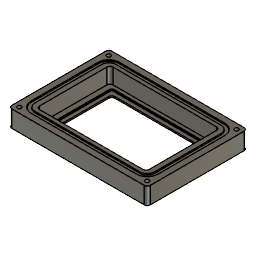
Base V3.4 (Autodesk Fusion 360 design; units mm, degrees)
part number: 2026-01-30-14-30-51-369
Autodesk Fusion 360 part; units mm, degrees
note: some values were not read from the file. Set by a fixed rule: which sketch regions a step uses.
sketch "Sketch1" plane through (0, 0, 0) normal (0, 0, 1) x (1, 0, 0)
  line L0 (86, -65) -> (-86, -65)
  line L1 (-90, -61) -> (-90, 61)
  line L2 (-86, 65) -> (86, 65)
  line L3 (90, 61) -> (90, -61)
  line L4 (90, -65) -> (-90, 65) construction
  line L5 (-90, -65) -> (90, 65) construction
  arc A0 (-86, 65) -> (-90, 61) centre (-86, 61) ccw
  arc A1 (90, 61) -> (86, 65) centre (86, 61) ccw
  arc A2 (86, -65) -> (90, -61) centre (86, -61) ccw
  arc A3 (-90, -61) -> (-86, -65) centre (-86, -61) ccw
  circle A4 centre (-83, 58) radius 2.6
  line L6 (0, 65) -> (0, -65) construction
  line L7 (90, 0) -> (-90, 0) construction
  circle A5 centre (83, 58) radius 2.6
  circle A6 centre (83, -58) radius 2.6
  circle A7 centre (-83, -58) radius 2.6
  dimension "d1" = 180
  dimension "d2" = 130
  dimension "d26" = 4
  dimension "d27" = 4
  dimension "d28" = 4
  dimension "d29" = 4
  dimension "d30" = 5.2
  dimension "d31" = 7
  dimension "d32" = 7
  constraint horizontal L0
  constraint perpendicular L0 L1
  constraint parallel L0 L2
  constraint parallel L1 L3
  constraint coincident L4 origin
  constraint coincident L5 origin
  constraint coincident L4.end L2
  constraint coincident L4.end L1
  constraint tangent L2 A0
  constraint tangent L1 A0
  constraint coincident L5.end L3
  constraint coincident L5.end L2
  constraint tangent L3 A1
  constraint tangent L2 A1
  constraint coincident L4.start L3
  constraint coincident L4.start L0
  constraint tangent L3 A2
  constraint tangent L0 A2
  constraint coincident L5.start L1
  constraint coincident L5.start L0
  constraint tangent L1 A3
  constraint tangent L0 A3
  constraint midpoint L2 L6.start
  constraint midpoint L0 L6.end
  constraint midpoint L3 L7.start
  constraint midpoint L1 L7.end
  constraint symmetric A4 L6 A5
  constraint symmetric A4 L7 A7
  constraint symmetric L7 A5 A6
  measures "d1" distance of L4.end L5.end
  measures "d2" distance of L5.start L4.end
  measures "d26" radius of A0
  measures "d27" radius of A1
  measures "d28" radius of A2
  measures "d29" radius of A3
  measures "d30" diameter of A4
  measures "d31" distance of L2 A4.centre
  measures "d32" distance of L1 A4.centre
extrude "Extrude1" add sketch "Sketch1" along normal blind 22
sketch "Sketch2" plane through (0, 0, 22) normal (0, 0, 1) x (-1, 0, 0)
  line L0 (-86, -65) -> (86, -65)
  line L1 (90, -61) -> (90, 61)
  line L2 (86, 65) -> (-86, 65)
  line L3 (-90, 61) -> (-90, -61)
  line L4 (-67.2, 47.75) -> (67.2, 47.75)
  line L5 (71.2, 43.75) -> (71.2, -43.75)
  line L6 (67.2, -47.75) -> (-67.2, -47.75)
  line L7 (-71.2, -43.75) -> (-71.2, 43.75)
  line L8 (-71.2, 47.75) -> (71.2, -47.75) construction
  line L9 (71.2, 47.75) -> (-71.2, -47.75) construction
  arc A0 (86, -65) -> (90, -61) centre (86, -61) ccw
  arc A1 (90, 61) -> (86, 65) centre (86, 61) ccw
  arc A2 (-86, 65) -> (-90, 61) centre (-86, 61) ccw
  arc A3 (-90, -61) -> (-86, -65) centre (-86, -61) ccw
  circle A4 centre (83, 58) radius 2.6
  circle A5 centre (-83, 58) radius 2.6
  circle A6 centre (-83, -58) radius 2.6
  circle A7 centre (83, -58) radius 2.6
  arc A8 (67.2, -47.75) -> (71.2, -43.75) centre (67.2, -43.75) ccw
  arc A9 (-71.2, -43.75) -> (-67.2, -47.75) centre (-67.2, -43.75) ccw
  arc A10 (71.2, 43.75) -> (67.2, 47.75) centre (67.2, 43.75) ccw
  arc A11 (-67.2, 47.75) -> (-71.2, 43.75) centre (-67.2, 43.75) ccw
  dimension "d5" = 142.4
  dimension "d6" = 95.5
  dimension "d52" = 4
  dimension "d53" = 4
  dimension "d54" = 4
  dimension "d55" = 4
  constraint horizontal L4
  constraint perpendicular L4 L5
  constraint parallel L4 L6
  constraint parallel L5 L7
  constraint coincident L8 origin
  constraint coincident L9 origin
  constraint coincident L8.end L6
  constraint coincident L8.end L5
  constraint tangent L6 A8
  constraint tangent L5 A8
  constraint coincident L9.end L6
  constraint coincident L9.end L7
  constraint tangent L6 A9
  constraint tangent L7 A9
  constraint coincident L9.start L5
  constraint coincident L9.start L4
  constraint tangent L5 A10
  constraint tangent L4 A10
  constraint coincident L8.start L7
  constraint coincident L8.start L4
  constraint tangent L7 A11
  constraint tangent L4 A11
  measures "d5" distance of L8.end L9.end
  measures "d6" distance of L9.start L8.end
  measures "d52" radius of A8
  measures "d53" radius of A9
  measures "d54" radius of A10
  measures "d55" radius of A11
extrude "Extrude2" cut sketch "Sketch2" against normal blind 20 contours L4 L5 L6 L7 A8 A9 A10 A11
sketch "Sketch3" plane through (0, 0, 22) normal (0, 0, 1) x (-1, 0, 0)
  line L0 (71.2, 43.75) -> (71.2, -43.75)
  line L1 (67.2, -47.75) -> (-67.2, -47.75)
  line L2 (-71.2, -43.75) -> (-71.2, 43.75)
  line L3 (-67.2, 47.75) -> (67.2, 47.75)
  line L4 (-86, -65) -> (86, -65)
  line L5 (90, -61) -> (90, 61)
  line L6 (86, 65) -> (-86, 65)
  line L7 (-90, 61) -> (-90, -61)
  line L8 (-79.9494, 54.9494) -> (79.9494, 54.9494) construction
  line L9 (79.9494, 54.9494) -> (79.9494, -54.9494) construction
  line L10 (79.9494, -54.9494) -> (-79.9494, -54.9494) construction
  line L11 (-79.9494, -54.9494) -> (-79.9494, 54.9494) construction
  line L12 (-79.9494, 54.9494) -> (79.9494, -54.9494) construction
  line L13 (79.9494, 54.9494) -> (-79.9494, -54.9494) construction
  line L14 (77.8149, 43.2459) -> (77.8149, -43.2459)
  line L15 (68.2459, -52.8149) -> (-68.2459, -52.8149)
  line L16 (-77.8149, -43.2459) -> (-77.8149, 43.2459)
  line L17 (-69.6267, 47.2574) -> (77.8149, -52.8149) construction
  line L18 (70.6619, 45.6619) -> (-70.6619, -45.6619) construction
  line L19 (-68.2459, 57.0839) -> (68.2459, 57.0839)
  line L20 (82.0839, 43.2459) -> (82.0839, -43.2459)
  line L21 (68.2459, -57.0839) -> (-68.2459, -57.0839)
  line L22 (-82.0839, -43.2459) -> (-82.0839, 43.2459)
  line L23 (-72.3401, 50.3077) -> (82.0839, -57.0839) construction
  line L24 (73.5309, 48.5309) -> (-73.5309, -48.5309) construction
  arc A0 (68.2459, -52.8149) -> (77.8149, -43.2459) centre (68.2459, -43.2459) ccw
  arc A1 (68.2459, -57.0839) -> (82.0839, -43.2459) centre (68.2459, -43.2459) ccw
  line L25 (0, -65) -> (0, 65) construction
  line L26 (-90, 0) -> (90, 0) construction
  arc A2 (-77.8149, -43.2459) -> (-68.2459, -52.8149) centre (-68.2459, -43.2459) ccw
  arc A3 (-82.0839, -43.2459) -> (-68.2459, -57.0839) centre (-68.2459, -43.2459) ccw
  arc A4 (-68.2459, 52.8149) -> (-77.8149, 43.2459) centre (-68.2459, 43.2459) ccw
  arc A5 (-68.2459, 57.0839) -> (-82.0839, 43.2459) centre (-68.2459, 43.2459) ccw
  arc A6 (77.8149, 43.2459) -> (68.2459, 52.8149) centre (68.2459, 43.2459) ccw
  arc A7 (82.0839, 43.2459) -> (68.2459, 57.0839) centre (68.2459, 43.2459) ccw
  line L27 (-68.2459, 52.8149) -> (68.2459, 52.8149)
  arc A8 (86, -65) -> (90, -61) centre (86, -61) ccw
  arc A9 (90, 61) -> (86, 65) centre (86, 61) ccw
  arc A10 (-86, 65) -> (-90, 61) centre (-86, 61) ccw
  arc A11 (-90, -61) -> (-86, -65) centre (-86, -61) ccw
  circle A12 centre (83, 58) radius 2.6
  circle A13 centre (-83, 58) radius 2.6
  circle A14 centre (-83, -58) radius 2.6
  circle A15 centre (83, -58) radius 2.6
  arc A16 (71.2, 43.75) -> (67.2, 47.75) centre (67.2, 43.75) ccw
  arc A17 (67.2, -47.75) -> (71.2, -43.75) centre (67.2, -43.75) ccw
  arc A18 (-71.2, -43.75) -> (-67.2, -47.75) centre (-67.2, -43.75) ccw
  arc A19 (-67.2, 47.75) -> (-71.2, 43.75) centre (-67.2, 43.75) ccw
  dimension "d9" = 159.8988
  dimension "d15" = 109.8988
  dimension "d16" = 2.1345
  dimension "d17" = 2.1345
  dimension "d18" = 2.1345
  dimension "d19" = 2.1345
  dimension "d20" = 9.569
  dimension "d21" = 13.838
  constraint horizontal L8
  constraint perpendicular L8 L9
  constraint parallel L8 L10
  constraint parallel L9 L11
  constraint coincident L12 origin
  constraint coincident L13 origin
  constraint parallel L15 L27
  constraint parallel L14 L16
  constraint coincident L17 origin
  constraint coincident L18 origin
  constraint horizontal L19
  constraint perpendicular L19 L20
  constraint parallel L19 L21
  constraint parallel L20 L22
  constraint coincident L23 origin
  constraint coincident L24 origin
  constraint coincident L17.end L15
  constraint coincident L17.end L14
  constraint tangent L15 A0
  constraint tangent L14 A0
  constraint coincident L23.end L21
  constraint coincident L23.end L20
  constraint tangent L21 A1
  constraint tangent L20 A1
  constraint midpoint L4 L25.start
  constraint midpoint L6 L25.end
  constraint midpoint L7 L26.start
  constraint midpoint L5 L26.end
  constraint symmetric L15.start L25 L15.end
  constraint symmetric L14.end L25 L16.start
  constraint symmetric A0 L25 A2
  constraint symmetric L21.start L25 L21.end
  constraint symmetric L20.end L25 L22.start
  constraint symmetric A1 L25 A3
  constraint symmetric L15.start L26 A6.end
  constraint symmetric L14.end L26 L14.start
  constraint symmetric A0 L26 A6
  constraint symmetric L21.start L26 L19.end
  constraint symmetric L20.end L26 L20.start
  constraint symmetric A1 L26 A7
  constraint symmetric L26 L15.end A4.start
  constraint symmetric L26 L16.start L16.end
  constraint symmetric L26 A2 A4
  constraint symmetric L26 L21.end L19.start
  constraint symmetric L26 L22.start L22.end
  constraint symmetric L26 A3 A5
  measures "d9" distance of L8.start L8.end
  measures "d15" distance of L8 L10
  measures "d16" distance of L11 L16
  measures "d17" distance of L10 L15
  measures "d18" distance of L11 L22
  measures "d19" distance of L10 L21
  measures "d20" radius of A0
  measures "d21" radius of A1
extrude "Extrude3" cut sketch "Sketch3" against normal blind 1.424 contours L19 L20 L21 L22 A1 A3 A5 A7
draft "Draft1" angle 10 neutral plane through (0, 0, 20.576) pull (0, 0, 1) 16 faces at (-77.8149, -14.4153, 21.5253) (-71.8024, 52.1295, 21.0507) (-22.7486, 52.8149, 21.5253) (72.6307, 51.7512, 21.0507) (77.8149, 14.4153, 21.5253) (73.0304, -51.5329, 21.0507) (22.7486, -52.8149, 21.5253) (-77.1295, -46.8024, 21.0507) (-82.0839, -14.4153, 21.5253) (-76.2727, -54.518, 21.0507) (-22.7486, -57.0839, 21.0507) (82.0213, -44.5613, 21.0507) (82.0839, 14.4153, 21.5253) (77.7952, 53.2609, 21.0507) (22.7486, 57.0839, 21.0507) (-76.8, 54.1233, 21.0507)
sketch "Sketch6" plane through (0, 0, 2) normal (0, 0, 1) x (-1, 0, 0)
  arc A0 (71.2, 43.75) -> (67.2, 47.75) centre (67.2, 43.75) ccw
  line L0 (67.2, 47.75) -> (-67.2, 47.75)
  arc A1 (-67.2, 47.75) -> (-71.2, 43.75) centre (-67.2, 43.75) ccw
  line L1 (-71.2, 43.75) -> (-71.2, -43.75)
  arc A2 (-71.2, -43.75) -> (-67.2, -47.75) centre (-67.2, -43.75) ccw
  line L2 (-67.2, -47.75) -> (67.2, -47.75)
  arc A3 (67.2, -47.75) -> (71.2, -43.75) centre (67.2, -43.75) ccw
  line L3 (71.2, -43.75) -> (71.2, 43.75)
  arc A4 (60.9079, -41.3399) -> (62.4799, -39.7679) centre (60.9079, -39.7679) ccw construction
  arc A5 (-62.4799, -39.7399) -> (-60.9079, -41.3119) centre (-60.9079, -39.7399) ccw construction
  line L4 (-48.9575, -41.8399) -> (48.9575, -41.8399) construction
  line L5 (48.9575, 41.8399) -> (-48.9575, 41.8399) construction
  line L6 (-62.9799, 29.7119) -> (-62.9799, 27.8175) construction
  line L7 (48.9575, -41.8399) -> (50.8519, -41.8399) construction
  line L8 (62.4799, 30.3078) -> (62.4799, 39.7679) construction
  arc A6 (-60.88, 42.74) -> (-63.88, 39.74) centre (-60.88, 39.74) ccw construction
  line L9 (63.88, 39.74) -> (63.88, -39.74) construction
  arc A7 (63.88, 39.74) -> (60.88, 42.74) centre (60.88, 39.74) ccw construction
  line L10 (-62.9799, -29.7119) -> (-62.4799, -30.3078) construction
  line L11 (51.4478, 41.3399) -> (50.8519, 41.8399) construction
  arc A8 (60.88, -42.74) -> (63.88, -39.74) centre (60.88, -39.74) ccw construction
  line L12 (-48.9575, 41.8399) -> (-50.8519, 41.8399) construction
  line L13 (-60.88, 42.74) -> (60.88, 42.74) construction
  line L14 (-62.9799, -27.8175) -> (-62.9799, -29.7119) construction
  line L15 (60.88, -42.74) -> (-60.88, -42.74) construction
  line L16 (62.9799, 29.7119) -> (62.4799, 30.3078) construction
  line L17 (-50.8519, 41.8399) -> (-51.4811, 41.3119) construction
  line L18 (62.4799, -39.7679) -> (62.4799, -30.3078) construction
  line L19 (-50.8519, -41.8399) -> (-48.9575, -41.8399) construction
  line L20 (60.9079, 41.3399) -> (51.4478, 41.3399) construction
  line L21 (50.8519, 41.8399) -> (48.9575, 41.8399) construction
  line L22 (62.9799, 27.8175) -> (62.9799, 29.7119) construction
  line L23 (51.4478, -41.3399) -> (60.9079, -41.3399) construction
  line L24 (62.9799, -27.8175) -> (62.9799, 27.8175) construction
  line L25 (-63.88, -39.74) -> (-63.88, 39.74) construction
  line L26 (50.8519, -41.8399) -> (51.4478, -41.3399) construction
  line L27 (62.9799, -29.7119) -> (62.9799, -27.8175) construction
  arc A9 (-63.88, -39.74) -> (-60.88, -42.74) centre (-60.88, -39.74) ccw construction
  arc A10 (62.4799, 39.7679) -> (60.9079, 41.3399) centre (60.9079, 39.7679) ccw construction
  line L28 (62.4799, -30.3078) -> (62.9799, -29.7119) construction
  line L29 (-62.4799, 30.3078) -> (-62.9799, 29.7119) construction
  line L30 (-60.9079, -41.3119) -> (-51.4811, -41.3119) construction
  arc A11 (-60.9079, 41.3119) -> (-62.4799, 39.7399) centre (-60.9079, 39.7399) ccw construction
  line L31 (-51.4811, -41.3119) -> (-50.8519, -41.8399) construction
  line L32 (-51.4811, 41.3119) -> (-60.9079, 41.3119) construction
  line L33 (-62.4799, 39.7399) -> (-62.4799, 30.3078) construction
  line L34 (-62.4799, -30.3078) -> (-62.4799, -39.7399) construction
  line L35 (-62.9799, 27.8175) -> (-62.9799, -27.8175) construction
  line L36 (0, -47.75) -> (0, 47.75) construction
  line L37 (-71.2, 0) -> (71.2, 0) construction
  line L38 (-60.85, 43.25) -> (60.85, 43.25)
  line L39 (64.35, 39.75) -> (64.35, -39.75)
  line L40 (60.85, -43.25) -> (-60.85, -43.25)
  line L41 (-64.35, -39.75) -> (-64.35, 39.75)
  line L42 (-64.35, 43.25) -> (64.35, -43.25) construction
  line L43 (64.35, 43.25) -> (-64.35, -43.25) construction
  arc A12 (60.85, -43.25) -> (64.35, -39.75) centre (60.85, -39.75) ccw
  arc A13 (-64.35, -39.75) -> (-60.85, -43.25) centre (-60.85, -39.75) ccw
  arc A14 (-60.85, 43.25) -> (-64.35, 39.75) centre (-60.85, 39.75) ccw
  arc A15 (64.35, 39.75) -> (60.85, 43.25) centre (60.85, 39.75) ccw
  line L44 (-60.85, 40.75) -> (60.85, 40.75)
  line L45 (61.85, 39.75) -> (61.85, -39.75)
  line L46 (60.85, -40.75) -> (-60.85, -40.75)
  line L47 (-61.85, -39.75) -> (-61.85, 39.75)
  line L48 (-61.85, 40.75) -> (61.85, -40.75) construction
  line L49 (61.85, 40.75) -> (-61.85, -40.75) construction
  arc A16 (-61.85, -39.75) -> (-60.85, -40.75) centre (-60.85, -39.75) ccw
  arc A17 (60.85, -40.75) -> (61.85, -39.75) centre (60.85, -39.75) ccw
  arc A18 (61.85, 39.75) -> (60.85, 40.75) centre (60.85, 39.75) ccw
  arc A19 (-60.85, 40.75) -> (-61.85, 39.75) centre (-60.85, 39.75) ccw
  dimension "d56" = 128.7
  dimension "d57" = 86.5
  dimension "d58" = 3.5
  dimension "d59" = 3.5
  dimension "d60" = 3.5
  dimension "d61" = 3.5
  dimension "d63" = 2.5
  dimension "d64" = 2.5
  dimension "d65" = 1
  dimension "d66" = 1
  dimension "d67" = 1
  dimension "d68" = 1
  constraint midpoint L2 L36.start
  constraint midpoint L0 L36.end
  constraint midpoint L1 L37.start
  constraint midpoint L3 L37.end
  constraint horizontal L38
  constraint perpendicular L38 L39
  constraint parallel L38 L40
  constraint parallel L39 L41
  constraint coincident L42 origin
  constraint coincident L43 origin
  constraint coincident L42.end L40
  constraint coincident L42.end L39
  constraint tangent L40 A12
  constraint tangent L39 A12
  constraint coincident L43.end L41
  constraint coincident L43.end L40
  constraint tangent L41 A13
  constraint tangent L40 A13
  constraint coincident L42.start L41
  constraint coincident L42.start L38
  constraint tangent L41 A14
  constraint tangent L38 A14
  constraint coincident L43.start L38
  constraint coincident L43.start L39
  constraint tangent L38 A15
  constraint tangent L39 A15
  constraint horizontal L44
  constraint perpendicular L44 L45
  constraint parallel L44 L46
  constraint parallel L45 L47
  constraint coincident L48 origin
  constraint coincident L49 origin
  constraint coincident L49.end L47
  constraint coincident L49.end L46
  constraint tangent L47 A16
  constraint tangent L46 A16
  constraint coincident L48.end L46
  constraint coincident L48.end L45
  constraint tangent L46 A17
  constraint tangent L45 A17
  constraint coincident L49.start L44
  constraint coincident L49.start L45
  constraint tangent L44 A18
  constraint tangent L45 A18
  constraint coincident L48.start L47
  constraint coincident L48.start L44
  constraint tangent L47 A19
  constraint tangent L44 A19
  measures "d56" distance of L42.end L43.end
  measures "d57" distance of L43.start L42.end
  measures "d58" radius of A12
  measures "d59" radius of A13
  measures "d60" radius of A14
  measures "d61" radius of A15
  measures "d63" distance of L41 L47
  measures "d64" distance of L40 L46
  measures "d65" radius of A16
  measures "d66" radius of A17
  measures "d67" radius of A18
  measures "d68" radius of A19
extrude "Extrude7" cut sketch "Sketch6" against normal blind 1 contours L38 L39 L40 L41 A12 A13 A14 A15
sketch "Sketch4" plane through (0, 0, 2) normal (0, 0, 1) x (-1, 0, 0)
  line L0 (-67.2, -47.75) -> (67.2, -47.75)
  line L1 (71.2, -43.75) -> (71.2, 43.75)
  line L2 (67.2, 47.75) -> (-67.2, 47.75)
  line L3 (-71.2, 43.75) -> (-71.2, -43.75)
  line L4 (-52.85, 35.75) -> (52.85, 35.75)
  line L5 (56.85, 31.75) -> (56.85, -31.75)
  line L6 (52.85, -35.75) -> (-52.85, -35.75)
  line L7 (-56.85, -31.75) -> (-56.85, 31.75)
  line L8 (-56.85, 35.75) -> (56.85, -35.75) construction
  line L9 (56.85, 35.75) -> (-56.85, -35.75) construction
  arc A0 (71.2, 43.75) -> (67.2, 47.75) centre (67.2, 43.75) ccw
  arc A1 (-67.2, 47.75) -> (-71.2, 43.75) centre (-67.2, 43.75) ccw
  arc A2 (-71.2, -43.75) -> (-67.2, -47.75) centre (-67.2, -43.75) ccw
  arc A3 (67.2, -47.75) -> (71.2, -43.75) centre (67.2, -43.75) ccw
  arc A4 (52.85, -35.75) -> (56.85, -31.75) centre (52.85, -31.75) ccw
  arc A5 (-56.85, -31.75) -> (-52.85, -35.75) centre (-52.85, -31.75) ccw
  arc A6 (-52.85, 35.75) -> (-56.85, 31.75) centre (-52.85, 31.75) ccw
  arc A7 (56.85, 31.75) -> (52.85, 35.75) centre (52.85, 31.75) ccw
  line L10 (64.35, 39.75) -> (64.35, -39.75)
  arc A8 (60.85, -43.25) -> (64.35, -39.75) centre (60.85, -39.75) ccw
  line L11 (60.85, -43.25) -> (-60.85, -43.25)
  arc A9 (-64.35, -39.75) -> (-60.85, -43.25) centre (-60.85, -39.75) ccw
  line L12 (-64.35, -39.75) -> (-64.35, 39.75)
  arc A10 (-60.85, 43.25) -> (-64.35, 39.75) centre (-60.85, 39.75) ccw
  line L13 (-60.85, 43.25) -> (60.85, 43.25)
  arc A11 (64.35, 39.75) -> (60.85, 43.25) centre (60.85, 39.75) ccw
  line L14 (61.85, -39.75) -> (61.85, 39.75)
  arc A12 (61.85, 39.75) -> (60.85, 40.75) centre (60.85, 39.75) ccw
  line L15 (60.85, 40.75) -> (-60.85, 40.75)
  arc A13 (-60.85, 40.75) -> (-61.85, 39.75) centre (-60.85, 39.75) ccw
  line L16 (-61.85, 39.75) -> (-61.85, -39.75)
  arc A14 (-61.85, -39.75) -> (-60.85, -40.75) centre (-60.85, -39.75) ccw
  line L17 (-60.85, -40.75) -> (60.85, -40.75)
  arc A15 (60.85, -40.75) -> (61.85, -39.75) centre (60.85, -39.75) ccw
  dimension "d71" = 4
  dimension "d72" = 4
  dimension "d73" = 4
  dimension "d74" = 4
  dimension "d77" = 5
  dimension "d78" = 5
  constraint horizontal L4
  constraint perpendicular L4 L5
  constraint parallel L4 L6
  constraint parallel L5 L7
  constraint coincident L8 origin
  constraint coincident L9 origin
  constraint coincident L8.end L6
  constraint coincident L8.end L5
  constraint tangent L6 A4
  constraint tangent L5 A4
  constraint coincident L9.end L6
  constraint coincident L9.end L7
  constraint tangent L6 A5
  constraint tangent L7 A5
  constraint coincident L8.start L7
  constraint coincident L8.start L4
  constraint tangent L7 A6
  constraint tangent L4 A6
  constraint coincident L9.start L4
  constraint coincident L9.start L5
  constraint tangent L4 A7
  constraint tangent L5 A7
  measures "d71" radius of A4
  measures "d72" radius of A5
  measures "d73" radius of A6
  measures "d74" radius of A7
  measures "d77" distance of L7 L16
  measures "d78" distance of L6 L17
extrude "Extrude8" cut sketch "Sketch4" against normal blind 5 contours L4 L5 L6 L7 A4 A5 A6 A7
equation "d9 = ( ORingPerimeter - 100 mm ) / 4 + 50 mm"
equation "ORingDiameter = 1.78 mm" comment "Diamter of the O ring"
equation "ORingInnerDiameter = 170 mm" comment "Inner diamter of the o ring bore"
equation "ORingPerimeter = 2 * 3.1412 * ( ( ORingInnerDiameter / 2 ) + ORingDiameter / 2 )"
equation "PanelWidth = 80 mm"
equation "PanelLength = 115 mm"
equation "d15 = ( ORingPerimeter - 100 mm ) / 4"
equation "d16 = ( ( ORingDiameter * 1.05 ) / 2 ) + 1.2 mm"
equation "d17 = ( ( ORingDiameter * 1.05 ) / 2 ) + 1.2 mm"
equation "d18 = ( ( ORingDiameter * 1.05 ) / 2 ) + 1.2 mm"
equation "d19 = ( ( ORingDiameter * 1.05 ) / 2 ) + 1.2 mm"
equation "d20 = ( ORingDiameter ) * 6 + ORingDiameter * 0.05 - 1.2 mm"
equation "d21 = ( ORingDiameter ) * 6 + ( ORingDiameter * 1.1 ) + 1.2 mm"
equation "d22 = -ORingDiameter * 0.8"
equation "d30 = Insert_OD - 0.5 mm"
equation "ORing2Diameter = 2 mm" comment "Second O ring Diameter"
equation "ORing2InnerDiameter = 126 mm" comment "Inner diameter of the second O Ring"
equation "ORing2Perimeter = 2 * 3.1412 * ( ( ORing2InnerDiameter / 2 ) + ORing2Diameter / 2 )"
equation "Bolt_Diam = 4 mm" comment "Diameter of the bolt"
equation "Bolt_Head_Height = 4 mm" comment "height of the bolt head"
equation "Bolt_Head_Diam = 7.22 mm" comment "Diameter of the bolt head"
equation "Insert_OD = 5.7 mm" comment "Outer Diameter of the insert"
